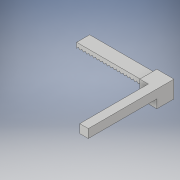
# Autodesk Inventor part: rackPart
Saved by Autodesk Inventor 2019 (Build 230136000, 136)
## iProperties
Created: 2018-11-15
Part Number: rackPart
Material: Generic
Document SubType Name: Modeling
Designer: Charlie
Density: 1 g/cm^3
Appearance: Default
Author: Charlie
Autodesk Inventor part; units mm, degrees
ref_plane "YZ Plane" through (0, 0, 0) normal (1, 0, 0) x (0, 1, 0)
ref_plane "XZ Plane" through (0, 0, 0) normal (0, 1, 0) x (-1, 0, 0)
ref_plane "XY Plane" through (0, 0, 0) normal (0, 0, 1) x (1, 0, 0)
sketch "Sketch1" plane through (0, 0, 0) normal (0, 0, 1) x (1, 0, 0)
  line L0 (-6.35, -6.35) -> (6.35, -6.35)
  line L1 (6.35, -6.35) -> (6.35, 6.35)
  line L2 (6.35, 6.35) -> (-6.35, 6.35)
  line L3 (-6.35, 6.35) -> (-6.35, -6.35)
  point P0 (0, 0)
  dimension "d0" = 12.7
  dimension "d1" = 12.7
  dimension "d2" = 6.35
  dimension "d3" = 6.35
  constraints: 8 end point, 2 parallel, 1 horizontal, 1 perpendicular
  measures "d0" distance of L2.end L1.end
  measures "d1" distance of L1.end L0.end
  measures "d2" distance from line of L2 point (0, 0)
  measures "d3" distance from line of L1 point (0, 0)
extrude "Extrusion1" add sketch "Sketch1" along normal blind 12.7
sketch "Sketch2" plane through (-6.35, -6.35, 0) normal (-1, 0, 0) x (0, 0, 1)
  point P0 (0, 6.35)
sketch "Sketch3" plane through (-6.35, -6.35, 0) normal (-1, 0, 0) x (0, 0, 1)
  line L0 (1.524, 11.43) -> (11.176, 11.43)
  line L1 (11.176, 11.43) -> (11.176, 7.62)
  line L2 (11.176, 7.62) -> (1.524, 7.62)
  line L3 (1.524, 7.62) -> (1.524, 11.43)
  line L4 (0, 12.7) -> (12.7, 12.7) projected
  line L5 (12.7, 12.7) -> (12.7, 0) projected
  line L6 (0, 12.7) -> (0, 0) projected
  point P0 (0, 6.35)
  dimension "d6" = 1.27
  dimension "d7" = 1.524
  dimension "d8" = 1.524
  dimension "d9" = 3.81
  constraints: 8 end point, 2 parallel, 1 horizontal, 1 perpendicular
  measures "d6" distance between parallel lines of L4 L0
  measures "d7" distance between parallel lines of L5 L1
  measures "d8" distance between parallel lines of L6 L3
  measures "d9" distance between parallel lines of L0 L2
extrude "Extrusion2" add sketch "Sketch3" along normal blind 48.26
sketch "Sketch4" plane through (0, 0, 12.7) normal (0, 0, 1) x (1, 0, 0)
  line L0 (6.35, -6.35) -> (6.35, 6.35) projected
  line L1 (0, 0) -> (6.35, 0)
  line L2 (6.35, 0) -> (6.35, 6.35)
  line L3 (6.35, 6.35) -> (0, 6.35)
  line L4 (0, 6.35) -> (0, 0)
  constraints: 8 end point, 2 parallel, 1 horizontal, 1 perpendicular
extrude "Extrusion3" add sketch "Sketch4" along normal blind 50.8
sketch "Sketch5" plane through (-6.35, 1.27, 11.176) normal (0, 0, 1) x (1, 0, 0)
  line L0 (0, 0) -> (-48.26, 0) projected
  line L1 (-46.99, 1.27) -> (-48.26, 0)
  line L2 (-46.99, 1.27) -> (-45.72, 0)
  line L3 (-48.26, 0) -> (-45.72, 0)
  line L4 (-44.45, 1.27) -> (-45.72, 0)
  line L5 (-45.72, 0) -> (-43.18, 0)
  line L6 (-44.45, 1.27) -> (-43.18, 0)
  line L7 (-41.91, 1.27) -> (-43.18, 0)
  line L8 (-43.18, 0) -> (-40.64, 0)
  line L9 (-41.91, 1.27) -> (-40.64, 0)
  line L10 (-39.37, 1.27) -> (-40.64, 0)
  line L11 (-40.64, 0) -> (-38.1, 0)
  line L12 (-39.37, 1.27) -> (-38.1, 0)
  line L13 (-36.83, 1.27) -> (-38.1, 0)
  line L14 (-38.1, 0) -> (-35.56, 0)
  line L15 (-36.83, 1.27) -> (-35.56, 0)
  line L16 (-34.29, 1.27) -> (-35.56, 0)
  line L17 (-35.56, 0) -> (-33.02, 0)
  line L18 (-34.29, 1.27) -> (-33.02, 0)
  line L19 (-31.75, 1.27) -> (-33.02, 0)
  line L20 (-33.02, 0) -> (-30.48, 0)
  line L21 (-31.75, 1.27) -> (-30.48, 0)
  line L22 (-29.21, 1.27) -> (-30.48, 0)
  line L23 (-30.48, 0) -> (-27.94, 0)
  line L24 (-29.21, 1.27) -> (-27.94, 0)
  line L25 (-26.67, 1.27) -> (-27.94, 0)
  line L26 (-27.94, 0) -> (-25.4, 0)
  line L27 (-26.67, 1.27) -> (-25.4, 0)
  line L28 (-24.13, 1.27) -> (-25.4, 0)
  line L29 (-25.4, 0) -> (-22.86, 0)
  line L30 (-24.13, 1.27) -> (-22.86, 0)
  line L31 (-21.59, 1.27) -> (-22.86, 0)
  line L32 (-22.86, 0) -> (-20.32, 0)
  line L33 (-21.59, 1.27) -> (-20.32, 0)
  line L34 (-19.05, 1.27) -> (-20.32, 0)
  line L35 (-20.32, 0) -> (-17.78, 0)
  line L36 (-19.05, 1.27) -> (-17.78, 0)
  line L37 (-16.51, 1.27) -> (-17.78, 0)
  line L38 (-17.78, 0) -> (-15.24, 0)
  line L39 (-16.51, 1.27) -> (-15.24, 0)
  line L40 (-13.97, 1.27) -> (-15.24, 0)
  line L41 (-15.24, 0) -> (-12.7, 0)
  line L42 (-13.97, 1.27) -> (-12.7, 0)
  line L43 (-11.43, 1.27) -> (-12.7, 0)
  line L44 (-12.7, 0) -> (-10.16, 0)
  line L45 (-11.43, 1.27) -> (-10.16, 0)
  line L46 (-8.89, 1.27) -> (-10.16, 0)
  line L47 (-10.16, 0) -> (-7.62, 0)
  line L48 (-8.89, 1.27) -> (-7.62, 0)
  line L49 (-6.35, 1.27) -> (-7.62, 0)
  line L50 (-7.62, 0) -> (-5.08, 0)
  line L51 (-6.35, 1.27) -> (-5.08, 0)
  line L52 (-3.81, 1.27) -> (-5.08, 0)
  line L53 (-5.08, 0) -> (-2.54, 0)
  line L54 (-3.81, 1.27) -> (-2.54, 0)
  line L55 (-1.27, 1.27) -> (-2.54, 0)
  line L56 (-2.54, 0) -> (0, 0)
  line L57 (-1.27, 1.27) -> (0, 0)
  point P0 (6.35, -1.27)
  dimension "d17" = 1.27
  dimension "d18" = 1.27
  dimension "d19" = 1.27
  dimension "d20" = 1.27
  dimension "d23" = 2.54
  constraints: 114 end point, 1 collinear, 1 horizontal, 1 point on line, 108 other
  measures "d17" distance from line of L0 L1.start
  measures "d18" horizontal distance of L1.start L2.end
  measures "d19" horizontal distance of L0.end L1.start
  measures "d20" horizontal distance of L1.start L0.end
  measures "d23" distance of L1.start L4.start
extrude "Extrusion4" cut sketch "Sketch5" against normal blind 50.8
body "Solid1"
